box (Autodesk Fusion 360 design; units mm, degrees)
Autodesk Fusion 360 part; units mm, degrees
note: some values were not read from the file. Set by a fixed rule: which sketch regions a step uses.
sketch "Sketch1" plane through (0, 0, 0) normal (1, 0, 0) x (0, 1, 0)
  line L0 (3.44, 4.5007) -> (-3.44, 4.5007)
  line L1 (2.3572, -10.2) -> (2.3572, -8)
  line L2 (5.2993, 8) -> (5.2993, 6.6428)
  line L3 (-8.2, 5.4993) -> (-6.56, 5.4993)
  line L4 (4.7007, 3.3572) -> (6.6428, 5.2993)
  line L5 (5.2993, -6.6428) -> (5.2993, -8)
  line L6 (-8.2, -5.4993) -> (-8.2, -2.84)
  line L7 (-5.4993, -6.56) -> (-3.44, -4.5007)
  line L8 (-3.3572, 4.7007) -> (-5.2993, 6.6428)
  line L9 (8, 2.3572) -> (10.2, 4.5572)
  line L10 (10, -10) -> (10, -4.64)
  line L11 (10.2, -2.3572) -> (8, -2.3572)
  line L12 (5.4993, 6.56) -> (3.44, 4.5007)
  line L13 (8.2, 2.84) -> (10, 4.64)
  line L14 (-5.2993, 6.6428) -> (-5.2993, 8)
  line L15 (-8.2, 2.84) -> (-8.2, 5.4993)
  line L16 (-6.6428, -5.2993) -> (-8, -5.2993)
  line L17 (-10, 4.64) -> (-8.2, 2.84)
  line L18 (10.2, 10.2) -> (4.5572, 10.2)
  line L19 (-4.5572, 10.2) -> (-10.2, 10.2)
  line L20 (3.3572, 4.7007) -> (-3.3572, 4.7007)
  line L21 (-10.2, 2.3572) -> (-10.2, 4.5572)
  line L22 (10, 4.64) -> (10, 10)
  line L23 (-2.3572, 10.2) -> (-2.3572, 8)
  line L24 (-8, 2.3572) -> (-10.2, 2.3572)
  line L25 (-2.3572, 8) -> (-4.5572, 10.2)
  line L26 (6.56, 5.4993) -> (8.2, 5.4993)
  line L27 (-2.84, -8.2) -> (-5.4993, -8.2)
  line L28 (8, 2.3572) -> (10.2, 2.3572)
  line L29 (4.5007, 3.44) -> (6.56, 5.4993)
  line L30 (2.3572, -8) -> (4.5572, -10.2)
  line L31 (10.2, 2.3572) -> (10.2, 4.5572)
  line L32 (2.84, 8.2) -> (5.4993, 8.2)
  line L33 (4.64, 10) -> (2.84, 8.2)
  line L34 (4.5572, 10.2) -> (2.3572, 8)
  line L35 (10.2, -4.5572) -> (10.2, -2.3572)
  line L36 (10, -4.64) -> (8.2, -2.84)
  line L37 (10.2, -10.2) -> (10.2, -4.5572)
  line L38 (-3.3572, -4.7007) -> (3.3572, -4.7007)
  line L39 (-3.44, -4.5007) -> (3.44, -4.5007)
  line L40 (5.4993, -8.2) -> (2.84, -8.2)
  line L41 (5.4993, -6.56) -> (5.4993, -8.2)
  line L42 (8, -5.2993) -> (6.6428, -5.2993)
  line L43 (4.7007, -3.3572) -> (4.7007, 3.3572)
  line L44 (6.6428, -5.2993) -> (4.7007, -3.3572)
  line L45 (5.2993, -8) -> (2.3572, -8)
  line L46 (4.5572, -10.2) -> (10.2, -10.2)
  circle A0 centre (0, 0) radius 2.5
  line L47 (-15, 15) -> (15, -15) construction
  line L48 (10.2, -4.5572) -> (8, -2.3572)
  line L49 (8.2, -5.4993) -> (6.56, -5.4993)
  line L50 (4.5007, -3.44) -> (4.5007, 3.44)
  line L51 (15, -15) -> (15, 15)
  line L52 (8.2, -2.84) -> (8.2, -5.4993)
  line L53 (4.5572, -10.2) -> (2.3572, -10.2)
  line L54 (-15, -15) -> (15, -15)
  line L55 (15, 15) -> (-15, 15)
  line L56 (4.64, -10) -> (10, -10)
  line L57 (6.56, -5.4993) -> (4.5007, -3.44)
  line L58 (-15, 15) -> (-15, -15)
  line L59 (3.3572, -4.7007) -> (5.2993, -6.6428)
  line L60 (2.84, -8.2) -> (4.64, -10)
  line L61 (8, -2.3572) -> (8, -5.2993)
  line L62 (3.44, -4.5007) -> (5.4993, -6.56)
  line L63 (15, 15) -> (-15, -15) construction
  line L64 (-8.2, -2.84) -> (-10, -4.64)
  line L65 (-8, 5.2993) -> (-6.6428, 5.2993)
  line L66 (-8, -5.2993) -> (-8, -2.3572)
  line L67 (-3.44, 4.5007) -> (-5.4993, 6.56)
  line L68 (-5.4993, -8.2) -> (-5.4993, -6.56)
  line L69 (-4.5007, 3.44) -> (-4.5007, -3.44)
  line L70 (-5.4993, 6.56) -> (-5.4993, 8.2)
  line L71 (-10, -4.64) -> (-10, -10)
  line L72 (-10.2, 4.5572) -> (-8, 2.3572)
  line L73 (10.2, 4.5572) -> (10.2, 10.2)
  line L74 (8, 5.2993) -> (8, 2.3572)
  line L75 (2.3572, 8) -> (5.2993, 8)
  line L76 (-8, -2.3572) -> (-10.2, -4.5572)
  line L77 (-5.2993, -6.6428) -> (-3.3572, -4.7007)
  line L78 (-4.5572, -10.2) -> (-2.3572, -8)
  line L79 (-8, -2.3572) -> (-10.2, -2.3572)
  line L80 (5.4993, 8.2) -> (5.4993, 6.56)
  line L81 (-2.3572, -10.2) -> (-4.5572, -10.2)
  line L82 (-2.84, 8.2) -> (-4.64, 10)
  line L83 (-10, -10) -> (-4.64, -10)
  line L84 (-8, 2.3572) -> (-8, 5.2993)
  line L85 (2.3572, 10.2) -> (4.5572, 10.2)
  line L86 (8.2, 5.4993) -> (8.2, 2.84)
  line L87 (-10, 10) -> (-10, 4.64)
  line L88 (-5.2993, 8) -> (-2.3572, 8)
  line L89 (-10.2, -2.3572) -> (-10.2, -4.5572)
  line L90 (-10.2, -4.5572) -> (-10.2, -10.2)
  line L91 (-6.56, -5.4993) -> (-8.2, -5.4993)
  line L92 (-4.64, 10) -> (-10, 10)
  line L93 (-5.4993, 8.2) -> (-2.84, 8.2)
  line L94 (-6.56, 5.4993) -> (-4.5007, 3.44)
  line L95 (-2.3572, -8) -> (-2.3572, -10.2)
  line L96 (-4.5007, -3.44) -> (-6.56, -5.4993)
  line L97 (-4.64, -10) -> (-2.84, -8.2)
  line L98 (-10.2, -10.2) -> (-4.5572, -10.2)
  line L99 (-5.2993, -8) -> (-5.2993, -6.6428)
  line L100 (6.6428, 5.2993) -> (8, 5.2993)
  line L101 (5.2993, 6.6428) -> (3.3572, 4.7007)
  line L102 (-2.3572, -8) -> (-5.2993, -8)
  line L103 (10, 10) -> (4.64, 10)
  line L104 (-6.6428, 5.2993) -> (-4.7007, 3.3572)
  line L105 (-4.7007, -3.3572) -> (-6.6428, -5.2993)
  line L106 (-4.5572, 10.2) -> (-2.3572, 10.2)
  line L107 (-4.7007, 3.3572) -> (-4.7007, -3.3572)
  line L108 (2.3572, 8) -> (2.3572, 10.2)
  line L109 (-10.2, 10.2) -> (-10.2, 4.5572)
  line L110 (0, 15) -> (66, 15)
  line L111 (66, 15) -> (66, 10)
  line L112 (66, 10) -> (15, 10)
  line L113 (0, 15) -> (-66, 15)
  line L114 (-66, 15) -> (-66, 10)
  line L115 (-66, 10) -> (-15, 10)
  line L116 (66, 15) -> (76, 15)
  line L117 (76, 15) -> (76, 10)
  line L118 (76, 10) -> (66, 10)
  line L119 (66, 10) -> (66, 15)
  line L120 (-66, 15) -> (-76, 15)
  line L121 (-76, 15) -> (-76, 10)
  line L122 (-76, 10) -> (-66, 10)
  line L123 (-66, 10) -> (-66, 15)
  line L124 (-2.3572, -10.2) -> (2.3572, -10.2)
  line L125 (0, -10.2) -> (0, -15)
  dimension "d143" = 0.2
  dimension "d2" = 30
  dimension "d3" = 30
  dimension "d13" = 5
  dimension "d5" = 66
  dimension "d6" = 5
  dimension "d7" = 66
  dimension "d8" = 5
  dimension "d9" = 10
  dimension "d10" = 5
  dimension "d11" = 10
  dimension "d12" = 5
  constraint parallel L88 L106
  constraint perpendicular L23 L88
  constraint perpendicular L24 L109
  constraint perpendicular L21 L24
  constraint perpendicular L75 L108
  constraint perpendicular L85 L108
  constraint perpendicular L28 L73
  constraint perpendicular L28 L31
  constraint parallel L35 L37
  constraint perpendicular L11 L37
  constraint parallel L46 L53
  constraint perpendicular L1 L45
  constraint perpendicular L95 L98
  constraint perpendicular L81 L95
  constraint perpendicular L79 L90
  constraint perpendicular L79 L89
  constraint horizontal L55
  constraint perpendicular L55 L58
  constraint parallel L54 L55
  constraint parallel L51 L58
  constraint coincident A0.centre L63
  constraint coincident A0.centre L47
  constraint coincident A0.centre origin
  constraint midpoint L55 L110.start
  constraint parallel L55 L110
  constraint perpendicular L110 L111
  constraint coincident L51 L112.end
  constraint perpendicular L51 L112
  constraint parallel L55 L113
  constraint perpendicular L113 L114
  constraint coincident L58 L115.end
  constraint perpendicular L58 L115
  constraint horizontal L116
  constraint vertical L117
  constraint horizontal L118
  constraint vertical L119
  constraint horizontal L120
  constraint vertical L121
  constraint horizontal L122
  constraint vertical L123
  constraint perpendicular L1 L124
  constraint midpoint L124 L125.start
  constraint midpoint L54 L125.end
  constraint perpendicular L54 L125
  measures "d2" distance of L54.start L47.end
  measures "d3" distance of L47.start L54.start
  measures "d13" diameter of A0
  measures "d5" distance of L110.start L110.end
  measures "d6" distance of L110.end L111.end
  measures "d7" distance of L110.start L113.end
  measures "d8" distance of L113.end L114.end
  measures "d9" distance of L110.end L116.end
  measures "d10" distance of L110.end L111.end
  measures "d11" distance of L113.end L120.end
  measures "d12" distance of L113.end L114.end
extrude "Extrude1" add sketch "Sketch1" along normal mid plane 20 contours L1 L5 L38 L45 L59 L77 L95 L99 L102 L124 | L51 L54 L55 L58 L110 L113 | L51 L110 L111 L112 L119 | L111 L116 L117 L118 L119 | L58 L113 L114 L115 L123 | L114 L120 L121 L122 L123
extrude "Extrude2" cut sketch "Sketch1" along normal mid plane 15 contours L1 L5 L38 L45 L59 L77 L95 L99 L102 L124
sketch "Sketch2" plane through (0, 0, -15) normal (0, 0, -1) x (1, 0, 0)
  line L0 (-10, -15) -> (10, -15)
  line L1 (10, -15) -> (10, 15)
  line L2 (10, 15) -> (-10, 15)
  line L3 (-10, 15) -> (-10, -15)
  circle A0 centre (0, 0) radius 2.5
  dimension "d18" = 5
  constraint coincident A0.centre origin
  measures "d18" diameter of A0
extrude "Extrude3" cut sketch "Sketch2" against normal blind 17 contours A0
sketch "Sketch3" plane through (0, 0, 15) normal (0, 0, 1) x (-1, 0, 0)
  line L0 (10, 76) -> (-10, 76)
  line L1 (-10, 76) -> (-10, -76)
  line L2 (-10, -76) -> (10, -76)
  line L3 (10, -76) -> (10, 76)
  circle A0 centre (0, 66) radius 2
  line L4 (0, 66) -> (0, 76)
  circle A1 centre (0, -66) radius 2
  line L5 (-10, 76) -> (10, 76)
  line L6 (10, 76) -> (10, 75)
  line L7 (10, 75) -> (-10, 75)
  line L8 (-10, 75) -> (-10, 76)
  line L9 (-10, -76) -> (10, -76)
  line L10 (10, -76) -> (10, -75)
  line L11 (10, -75) -> (-10, -75)
  line L12 (-10, -75) -> (-10, -76)
  point P0 (0, -66)
  dimension "d21" = 4
  dimension "d22" = 4
  dimension "d25" = 1
  dimension "d26" = 20
  dimension "d27" = 1
  constraint coincident A0.centre L4
  constraint coincident P0 A1.centre
  constraint horizontal L5
  constraint vertical L6
  constraint horizontal L7
  constraint vertical L8
  constraint coincident L0.end L1.start
  constraint horizontal L9
  constraint vertical L10
  constraint horizontal L11
  constraint vertical L12
  constraint coincident L1.end L2.start
  measures "d21" diameter of A0
  measures "d22" diameter of A1
  measures "d25" distance of L0.end L7.end
  measures "d26" distance of L1.end L2.end
  measures "d27" distance of L1.end L11.end
extrude "Extrude4" cut sketch "Sketch3" against normal blind 20 contours A0 | A1
fillet "Fillet2" radius 2 2 edges at (0, 76, 10) (0, -76, 10)
fillet "Fillet3" radius 20 2 edges at (0, -15, 10) (0, 15, 10)
fillet "Fillet4" radius 5 2 edges at (0, 15, -15) (0, -15, -15)
equation "d5 = ( 132 / 2 ) * 1 mm"
